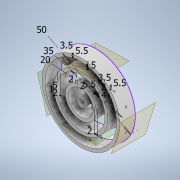
# Autodesk Inventor part: improved_gimbal
Saved by Autodesk Inventor 2021 (Build 250183000, 183)
## iProperties
Created: 2021-06-15
Part Number: improved_gimbal
Material: Generic
Document SubType Name: Modeling
Designer: Charlie
Density: 1 g/cm^3
Appearance: Default
Author: Charlie
Autodesk Inventor part; units mm, degrees
ref_plane "YZ Plane" through (0, 0, 0) normal (1, 0, 0) x (0, 1, 0)
ref_plane "XZ Plane" through (0, 0, 0) normal (0, 1, 0) x (-1, 0, 0)
ref_plane "XY Plane" through (0, 0, 0) normal (0, 0, 1) x (1, 0, 0)
sketch "Sketch1" plane through (0, 0, 0) normal (0, 0, 1) x (1, 0, 0)
  circle A0 centre (0, 0) radius 25
  circle A1 centre (0, 0) radius 23
  circle A2 centre (0, 0) radius 17.5
  circle A3 centre (0, 0) radius 15.5
  circle A4 centre (0, 0) radius 10
  circle A5 centre (0, 0) radius 8
  circle A6 centre (0, 0) radius 5
  line L0 (-0.4916, -7.9849) -> (0.4916, 7.9849) construction
  line L1 (0.4916, -7.9849) -> (-0.4916, 7.9849) construction
  circle A7 centre (0, 0) radius 2
  line L2 (-1, 7.9373) -> (-1, 4.899)
  line L3 (-1, -4.899) -> (-1, -7.9373)
  line L4 (1, -7.9373) -> (1, -4.899)
  line L5 (1, 4.899) -> (1, 7.9373)
  circle A8 centre (0, 0) radius 2.75
  circle A9 centre (10, 8.6308) radius 2.75
  circle A10 centre (10, 8.6308) radius 1.75
  circle A11 centre (-14.5742, 14.326) radius 2.75
  circle A12 centre (-14.5742, 14.326) radius 1.75
  point P0 (-23.9869, -7.0447)
  point P1 (23.9106, -7.2995)
  point P2 (-0.7169, 22.9888)
  point P3 (-0.308, -17.4973)
  point P4 (-0.6761, 17.4869)
  point P5 (-17.125, 15.3536)
  point P6 (-15.6456, 16.8587)
  point P7 (10.592, 11.3164)
  point P8 (12.7432, 8.8239)
  dimension "d0" = 50
  dimension "d1" = 2
  dimension "d2" = 35
  dimension "d3" = 2
  dimension "d4" = 20
  dimension "d5" = 2
  dimension "d16" = 4
  dimension "d17" = 2
  dimension "d18" = 2
  dimension "d19" = 5.5
  dimension "d58" = 5.5
  dimension "d59" = 3.5
  dimension "d60" = 5.5
  dimension "d61" = 3.5
  constraints: 12 end point, 11 centre point, 8 point on circle, 7 coincident, 4 parallel, 2 midpoint, 13 other
  measures "d0" diameter of A0
  measures "d2" diameter of A2
  measures "d3" radial gap between concentric circles of A2 A3
  measures "d4" diameter of A4
  measures "d16" diameter of A7
  measures "d17" distance between parallel lines of L4 L3
  measures "d18" distance between parallel lines of L2 L5
  measures "d19" diameter of A8
  measures "d58" diameter of A9
  measures "d59" diameter of A10
  measures "d60" diameter of A11
  measures "d61" diameter of A12
extrude "Extrusion1" add sketch "Sketch1" along normal blind 10 contours A0 | A1 A11 picked at (-16.4455, 16.1655)
ref_plane "Work Plane1" through (-23.9869, -7.0447, 0) normal (-0.9595, -0.2818, 0) x (0.2818, -0.9595, 0)
sketch "Sketch2" plane through (-23.9869, -7.0447, 0) normal (-0.9595, -0.2818, 0) x (0.2818, -0.9595, 0)
  line L0 (0, 0) -> (0, 5)
  circle A0 centre (0, 5) radius 0.5
  dimension "d22" = 5
  dimension "d23" = 1
  constraints: 2 end point, 1 centre point, 1 coincident, 1 vertical
  measures "d22" distance of L0.start L0.end
  measures "d23" diameter of A0
extrude "Extrusion2" cut sketch "Sketch2" against normal blind 50
extrude "Extrusion3" add sketch "Sketch1" along normal blind 10 contours A2 | A3 A9 picked at (11.845, 10.2232)
ref_plane "Work Plane2" through (-0.6761, 17.4869, 0) normal (-0.0386, 0.9993, 0) x (-0.9993, -0.0386, 0)
sketch "Sketch3" plane through (-0.6761, 17.4869, 0) normal (-0.0386, 0.9993, 0) x (-0.9993, -0.0386, 0)
  line L0 (0, 0) -> (0, 5)
  circle A0 centre (0, 5) radius 0.5
  dimension "d28" = 5
  dimension "d29" = 1
  constraints: 2 end point, 1 centre point, 1 coincident, 1 vertical
  measures "d28" distance of L0.start L0.end
  measures "d29" diameter of A0
extrude "Extrusion4" cut sketch "Sketch3" against normal blind 44
extrude "Extrusion5" cut sketch "Sketch2" against normal blind 4.5
ref_plane "Work Plane3" through (23.9106, -7.2995, 0) normal (0.9564, -0.292, 0) x (0.292, 0.9564, 0)
sketch "Sketch4" plane through (23.9106, -7.2995, 0) normal (0.9564, -0.292, 0) x (0.292, 0.9564, 0)
  circle A0 centre (0, 5) radius 0.5 projected
  circle A1 centre (0, 5) radius 0.5
  point P0 (0, 0)
  dimension "d34" = 1
  constraints: 1 centre point, 1 coincident
  measures "d34" diameter of A1
extrude "Extrusion6" cut sketch "Sketch4" against normal blind 4.5
extrude "Extrusion7" add sketch "Sketch1" along normal blind 10 contours A4
extrude "Extrusion8" cut sketch "Sketch3" against normal blind 5
ref_plane "Work Plane4" through (-0.308, -17.4973, 0) normal (-0.0176, -0.9998, 0) x (0.9998, -0.0176, 0)
sketch "Sketch5" plane through (-0.308, -17.4973, 0) normal (-0.0176, -0.9998, 0) x (0.9998, -0.0176, 0)
  circle A0 centre (0, 5) radius 0.5 projected
  circle A1 centre (0, 5) radius 0.5
  point P0 (0, 0)
  dimension "d41" = 1
  constraints: 1 centre point, 1 coincident
  measures "d41" diameter of A1
extrude "Extrusion9" cut sketch "Sketch5" against normal blind 5
extrude "Extrusion10" add sketch "Sketch1" along normal blind 2 contours L5 A6 L2 A5 | A5 L3 A6 L4 | A6
extrude "Extrusion11" add sketch "Sketch1" along normal blind 10 contours A8
extrude "Extrusion12" add sketch "Sketch1" along normal blind 5 contours A11 A1 | A9 A3 picked at (-15.6648, 16.3977) picked at (10.86, 10.7068)
body "Solid1"
